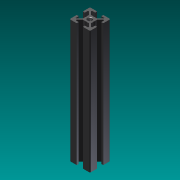
# Autodesk Inventor part: HFSY5-2020-120-TPW
Saved by Autodesk Inventor 2015 (Build 190159000, 159)
## iProperties
Category: PARTsolutions
Company: MISUMI
Created: 2016-02-29
Part Number: HFSY5-2020-120-TPW
Catalog Web Link: www.cadenas.de
Description: NFS5-2020, NFSB5-2020, HFS5-2020, HFSB5-2020, CAF5-2020, HFSY5-2020, NFSF5-2020, HFSF5-2020, HFSFB5-2020, NFST5-2020, HFST5-2020, HFSTB5-2020, HFSH5-2020, HFSC5-2020-HFS5 Series Aluminum Extrusions 20 Square -1 Slot-
Vendor: MISUMI
Document SubType Name: Modeling
Designer: psAdmin
Manufacturer: MISUMI
Mass: 21.8665 g
Surface Area: 212.07 cm^2
Volume: 21.8665 cm^3
Density: 1 g/cm^3
Material: 一般
Appearance: PSOLRGB-175-175-175
PSOL_IDENT_0: {$CADENAS_DATA\23d-libs\misumi\metric\38_al_extrusions_blackets\5\hfs5_2020.prj},580 {VTYP=3D},{NB=H
PSOL_IDENT_1: FSY5-2020-120-TPW},{LINA=HFSY5-2020-120-TPW},{NN=NFS5-2020, NFSB5-2020, HFS5-2020, HFSB5-2020, CAF5-
PSOL_IDENT_2: 2020, HFSY5-2020, NFSF5-2020, HFSF5-2020, HFSFB5-2020, NFST5-2020, HFST5-2020, HFSTB5-2020, HFSH5-20
PSOL_IDENT_3: 20, HFSC5-2020},{DATE=17.07.2015 10:47:07},{GEOMDATE=28.10.2014 00:00:00},{VERSION=},{LINEID=120},{L
PSOL_IDENT_4: INESUBID=-1},{WBVAR=L,ALT1,ALT2,ALT4,ALT5,CP5,DL5,DR5,ALT6,ALT9,ALT10,ALT11,HP6,NHL6,DL6,NHR6,DR6,AL
PSOL_IDENT_5: T7,ALT8,NH9,AH,BH,CH,DH,EH,NH10,AV,BV,CV,DV,EV,NH11,AP,BP,CP,DP,EP,ALT12,ALT13,Z,NH12,XA,XB,XC,XD,XE
PSOL_IDENT_6: ,NH13,YA,YB,YC,YD,YE,ALT16,HP16,DL16,DR16,ALT17,HQ17,JLP,ALT20}  {NB=HFSY5-2020-120-TPW},{LINA=HFSY5
PSOL_IDENT_7: -2020-120-TPW},{KT=DUMMY},{PN=HFSY5-2020-120-TPW},{TPS=HFSY5-2020},{MAT=A6N01SS-T5 Aluminum Alloy or
PSOL_IDENT_8: 6005A-T5 Aluminum Alloy},{ST=Baked-on Finish (Yellow)},{FRMW=20},{FRMH=20},{FRD=4.2},{L=120},{MASS=
PSOL_IDENT_9: 0.5},{SA=183},{LX=0.742x10^4},{LY=0.742x10^4},{ALT1=TPW},{M1=5},{DPL1=15},{DPR1=15},{ALT1PN=-TPW},{A
PSOL_IDENT_10: LT2=},{ALT2ALG= '','Not applicable' },{M2=0},{DP2=0},{ALT2PN=},{ALT4=},{ALT4ALG= '', 'w/o SC (High P
PSOL_IDENT_11: recision Cut)', 'SC', 'with SC (High Precision Cut)' },{ALT4PN=},{ALT5=},{ALT5ALG= '','w/o 45 Degree
PSOL_IDENT_12: Cut','1','with 45 Degree Cut' },{CP5=},{CP5ALG= '','N/A' },{DL5=},{DL5ALG= '','N/A' },{DR5=},{DR5AL
PSOL_IDENT_13: G= '','N/A' },{FRMLALT5=0},{FRMRALT5=0},{ALT5PN=},{ALT6=},{ALT6ALG= '','w/o Fastening Location Wrenc
PSOL_IDENT_14: h Access Hole Alterations','1','with Fastening Location Wrench Access Hole Alterations' },{ALT9=},{A
PSOL_IDENT_15: LT9ALG= '','w/o Location Specified Wrench Access Hole Alteratons (Horizontal)','1','with Location Sp
PSOL_IDENT_16: ecified Wrench Access Hole Alteratons (Horizontal)' },{ALT10=},{ALT10ALG= '','w/o Location Specified
PSOL_IDENT_17: Wrench Access Hole Alteratons (Vertical)','1','with Location Specified Wrench Access Hole Alteraton
PSOL_IDENT_18: s (Vertical)' },{ALT11=},{ALT11ALG= '','w/o Location Specified Wrench Access Hole Alteratons (Crissc
PSOL_IDENT_19: ross)','1','with Location Specified Wrench Access Hole Alteratons (Crisscross)' },{HP6=},{HP6ALG= ''
PSOL_IDENT_20: ,'N/A' },{NHL6=},{NHL6ALG= '','N/A' },{DL6=},{DL6ALG= '','N/A' },{NHR6=},{NHR6ALG= '','N/A' },{DR6=}
PSOL_IDENT_21: ,{DR6ALG= '','N/A' },{HL6=0},{HL6D=0},{HR6=0},{HR6D=0},{J6=0},{J6D=0},{K6=0},{K6D=0},{DD6=0.00},{DD6
PSOL_IDENT_22: ALG=0},{ALT7=},{ALT7ALG= '','N/A' },{ALT8=},{ALT8ALG= '','N/A' },{ALT678PN=},{NH9=0},{NH9MAX=5},{NH9
PSOL_IDENT_23: ALG=[0]},{AH=0.0},{AHMIN=7},{AHMAX=115},{AHALG=[0]},{BH=0.0},{BHMIN=2},{BHMAX=117},{BHALG=[0]},{CH=0
PSOL_IDENT_24: .0},{CHMIN=2},{CHMAX=119},{CHALG=[0]},{DH=0.0},{DHMIN=2},{DHMAX=121},{DHALG=[0]},{EH=0.0},{EHMIN=2},
PSOL_IDENT_25: {EHMAX=113},{EHALG=[0]},{NH10=0},{NH10MAX=5},{NH10ALG=[0]},{AV=0.0},{AVMIN=7},{AVMAX=115},{AVALG=[0]
PSOL_IDENT_26: },{BV=0.0},{BVMIN=2},{BVMAX=117},{BVALG=[0]},{CV=0.0},{CVMIN=2},{CVMAX=119},{CVALG=[0]},{DV=0.0},{DV
PSOL_IDENT_27: MIN=2},{DVMAX=121},{DVALG=[0]},{EV=0.0},{EVMIN=2},{EVMAX=113},{EVALG=[0]},{NH11=0},{NH11MAX=5},{NH11
PSOL_IDENT_28: ALG=[0]},{AP=0.0},{APMIN=7},{APMAX=115},{APALG=[0]},{BP=0.0},{BPMIN=2},{BPMAX=117},{BPALG=[0]},{CP=0
PSOL_IDENT_29: .0},{CPMIN=2},{CPMAX=119},{CPALG=[0]},{DP=0.0},{DPMIN=2},{DPMAX=121},{DPALG=[0]},{EP=0.0},{EPMIN=2},
PSOL_IDENT_30: {EPMAX=113},{EPALG=[0]},{ALT9PN=},{ALT10PN=},{ALT11PN=},{ALT91011PN=},{ALT12=},{ALT12ALG= '','w/o Co
PSOL_IDENT_31: unterbore Hole in Specified Position (Vertical)','1','with Counterbore Hole in Specified Position (V
PSOL_IDENT_32: ertical)' },{ALT13=},{ALT13ALG= '','w/o Counterbore Hole in Specified Position (Horizontal)','1','wi
PSOL_IDENT_33: th Counterbore Hole in Specified Position (Horizontal)' },{Z=},{ZALG= '','N/A' },{DD12=0.0},{DD112=0
PSOL_IDENT_34: .0},{NH12=0},{NH12MAX=5},{NH12ALG=[0]},{XA=0.0},{XAMIN=7},{XAMAX=115},{XAALG=[0]},{XB=0.0},{XBMIN=2}
PSOL_IDENT_35: ,{XBMAX=117},{XBALG=[0]},{XC=0.0},{XCMIN=2},{XCMAX=119},{XCALG=[0]},{XD=0.0},{XDMIN=2},{XDMAX=121},{
PSOL_IDENT_36: XDALG=[0]},{XE=0.0},{XEMIN=2},{XEMAX=113},{XEALG=[0]},{NH13=0},{NH13MAX=5},{NH13ALG=[0]},{YA=0.0},{Y
PSOL_IDENT_37: AMIN=7},{YAMAX=115},{YAALG=[0]},{YB=0.0},{YBMIN=2},{YBMAX=117},{YBALG=[0]},{YC=0.0},{YCMIN=2},{YCMAX=
PSOL_IDENT_38: 119},{YCALG=[0]},{YD=0.0},{YDMIN=2},{YDMAX=121},{YDALG=[0]},{YE=0.0},{YEMIN=2},{YEMAX=113},{YEALG=[0
PSOL_IDENT_39: ]},{ALT12PN=},{ALT13PN=},{ALT1213PN=},{ALT16=},{ALT16ALG= '','w/o M Type Hole Alteration','1','with
PSOL_IDENT_40: M Type Hole Alteration' },{HP16=},{HP16ALG= '','N/A' },{DL16=},{DL16ALG= '','N/A' },{DR16=},{DR16ALG=
PSOL_IDENT_41: '','N/A' },{H116=0},{D16=0.0},{ALT16PN=},{ALT17=},{ALT17ALG= '','w/o L Type Hole Alteration (Top)','
PSOL_IDENT_42: 1','with L Type Hole Alteration (Top)' },{HQ17=0},{HQ17ALG=0},{JLP=0},{JLPMIN=4.9},{JLPMAX=0},{JLPAL
PSOL_IDENT_43: G=[0]},{L17=0},{D17=0.0},{ALT17PN=},{ALT20=},{ALT20PN=},{ERRORALT01=OK},{ERRORALT02=OK},{ERRORALT05=
PSOL_IDENT_44: OK},{ERRORALT06091=OK},{ERRORALT06092=OK},{ERRORALT06093=OK},{ERRORALT06094=OK},{ERRORALT06101=OK},{
PSOL_IDENT_45: ERRORALT06102=OK},{ERRORALT06103=OK},{ERRORALT06104=OK},{ERRORALT06111=OK},{ERRORALT06112=OK},{ERROR
PSOL_IDENT_46: ALT06113=OK},{ERRORALT06114=OK},{ERRORALT06121=OK},{ERRORALT06122=OK},{ERRORALT06123=OK},{ERRORALT06
PSOL_IDENT_47: 124=OK},{ERRORALT06131=OK},{ERRORALT06132=OK},{ERRORALT06133=OK},{ERRORALT06134=OK},{ERRORALT0616=OK
PSOL_IDENT_48: },{ERRORALT06171=OK},{ERRORALT06172=OK},{ERRORALT06173=OK},{ERRORALT0911=OK},{ERRORALT0913=OK},{ERRO
PSOL_IDENT_49: RALT0916=OK},{ERRORALT0917=OK},{ERRORALT1011=OK},{ERRORALT1012=OK},{ERRORALT1016=OK},{ERRORALT1017=O
PSOL_IDENT_50: K},{ERRORALT1112=OK},{ERRORALT1113=OK},{ERRORALT1116=OK},{ERRORALT1117=OK},{ERRORALT1216=OK},{ERRORA
PSOL_IDENT_51: LT1217=OK},{ERRORALT1316=OK},{ERRORALT1317=OK},{ERRORALT1617=OK},{ERRORPN=},{TFW=0}
NN: NFS5-2020, NFSB5-2020, HFS5-2020, HFSB5-2020, CAF5-2020, HFSY5-2020, NFSF5-2020, HFSF5-2020, HFSFB5-2020, NFST5-2020, HFST5-2020, HFSTB5-2020, HFSH5-2020, HFSC5-2020
NT: HFS5 Series Aluminum Extrusions 20 Square -1 Slot-
NB: HFSY5-2020-120-TPW
NBSYN: $PN.
LINA: HFSY5-2020-120-TPW
PN: HFSY5-2020-120-TPW
TPS: HFSY5-2020
MAT: A6N01SS-T5 Aluminum Alloy or 6005A-T5 Aluminum Alloy
ST: Baked-on Finish (Yellow)
L: 120
MASS: 0.5
SA: 183
LX: 0.742x10^4
LY: 0.742x10^4
ALT1: with TPW (Tapping on Both Ends)
M1: 5
DPL1: 15
DPR1: 15
ALT2: Not applicable
M2: 0
DP2: 0
ALT4: w/o SC (High Precision Cut)
ALT5: w/o 45 Degree Cut
CP5: N/A
DL5: N/A
DR5: N/A
ALT6: w/o Fastening Location Wrench Access Hole Alterations
ALT9: w/o Location Specified Wrench Access Hole Alteratons (Horizontal)
ALT10: w/o Location Specified Wrench Access Hole Alteratons (Vertical)
ALT11: w/o Location Specified Wrench Access Hole Alteratons (Crisscross)
HP6: N/A
NHL6: N/A
DL6: N/A
NHR6: N/A
DR6: N/A
HL6D: 0
HR6D: 0
J6D: 0
K6D: 0
DD6: 0.00
ALT7: N/A
ALT8: N/A
NH9: 0
AH: 0.0
BH: 0.0
CH: 0.0
DH: 0.0
EH: 0.0
NH10: 0
AV: 0.0
BV: 0.0
CV: 0.0
DV: 0.0
EV: 0.0
NH11: 0
AP: 0.0
BP: 0.0
CP: 0.0
DP: 0.0
EP: 0.0
ALT12: w/o Counterbore Hole in Specified Position (Vertical)
ALT13: w/o Counterbore Hole in Specified Position (Horizontal)
Z: N/A
DD12: 0.0
DD112: 0.0
NH12: 0
XA: 0.0
XB: 0.0
XC: 0.0
XD: 0.0
XE: 0.0
NH13: 0
YA: 0.0
YB: 0.0
YC: 0.0
YD: 0.0
YE: 0.0
ALT16: w/o M Type Hole Alteration
HP16: N/A
DL16: N/A
DR16: N/A
H116: 0
D16: 0.0
ALT17: w/o L Type Hole Alteration (Top)
HQ17: 0
JLP: 0
D17: 0.0
ALT20: w/o CW (End Face C Chamfering)
SUPPLIER: MISUMI
ARTICLENO: HFSY5-2020-120-TPW
BOMINFO: HFSY5-2020-120-TPW
CREATOR: CADENAS GmbH
Title: HFSY5-2020-120-TPW
Author: Cadenas PARTsolutions
Comments: HFS5 Series Aluminum Extrusions 20 Square -1 Slot-
Autodesk Inventor part; units mm, degrees
sketch "Sketch_1" plane through (0, 0, 0) normal (0, 0, 1) x (1, 0, 0)
  line L0 (-10, 3) -> (-8, 3)
  line L1 (-8, 3) -> (-8, 6)
  line L2 (-8, 6) -> (-7.0607, 6)
  line L3 (-7.0607, 6) -> (-4, 2.9393)
  line L4 (-4, 2.9393) -> (-4, 0.5196)
  line L5 (-4, 0.5196) -> (-3.7, 0)
  line L6 (-3.7, 0) -> (-4, -0.5196)
  line L7 (-4, -0.5196) -> (-4, -2.9393)
  line L8 (-4, -2.9393) -> (-7.0607, -6)
  line L9 (-7.0607, -6) -> (-8, -6)
  line L10 (-8, -6) -> (-8, -3)
  line L11 (-8, -3) -> (-10, -3)
  line L12 (-10, -3) -> (-10, -9)
  arc A0 (-10, -9) -> (-9, -10) centre (-9, -9) ccw
  line L13 (-9, -10) -> (-3, -10)
  line L14 (-3, -10) -> (-3, -8)
  line L15 (-3, -8) -> (-6, -8)
  line L16 (-6, -8) -> (-6, -7.0607)
  line L17 (-6, -7.0607) -> (-2.9393, -4)
  line L18 (-2.9393, -4) -> (-0.5196, -4)
  line L19 (-0.5196, -4) -> (0, -3.7)
  line L20 (0, -3.7) -> (0.5196, -4)
  line L21 (0.5196, -4) -> (2.9393, -4)
  line L22 (2.9393, -4) -> (6, -7.0607)
  line L23 (6, -7.0607) -> (6, -8)
  line L24 (6, -8) -> (3, -8)
  line L25 (3, -8) -> (3, -10)
  line L26 (3, -10) -> (9, -10)
  arc A1 (9, -10) -> (10, -9) centre (9, -9) ccw
  line L27 (10, -9) -> (10, -3)
  line L28 (10, -3) -> (8, -3)
  line L29 (8, -3) -> (8, -6)
  line L30 (8, -6) -> (7.0607, -6)
  line L31 (7.0607, -6) -> (4, -2.9393)
  line L32 (4, -2.9393) -> (4, -0.5196)
  line L33 (4, -0.5196) -> (3.7, 0)
  line L34 (3.7, 0) -> (4, 0.5196)
  line L35 (4, 0.5196) -> (4, 2.9393)
  line L36 (4, 2.9393) -> (7.0607, 6)
  line L37 (7.0607, 6) -> (8, 6)
  line L38 (8, 6) -> (8, 3)
  line L39 (8, 3) -> (10, 3)
  line L40 (10, 3) -> (10, 9)
  arc A2 (10, 9) -> (9, 10) centre (9, 9) ccw
  line L41 (9, 10) -> (3, 10)
  line L42 (3, 10) -> (3, 8)
  line L43 (3, 8) -> (6, 8)
  line L44 (6, 8) -> (6, 7.0607)
  line L45 (6, 7.0607) -> (2.9393, 4)
  line L46 (2.9393, 4) -> (0.5196, 4)
  line L47 (0.5196, 4) -> (0, 3.7)
  line L48 (0, 3.7) -> (-0.5196, 4)
  line L49 (-0.5196, 4) -> (-2.9393, 4)
  line L50 (-2.9393, 4) -> (-6, 7.0607)
  line L51 (-6, 7.0607) -> (-6, 8)
  line L52 (-6, 8) -> (-3, 8)
  line L53 (-3, 8) -> (-3, 10)
  line L54 (-3, 10) -> (-9, 10)
  arc A3 (-9, 10) -> (-10, 9) centre (-9, 9) ccw
  line L55 (-10, 9) -> (-10, 3)
  constraints: 112 end point, 8 point on circle, 4 centre point
extrude "Extrusion1" add sketch "Sketch_1" against normal blind 120
sketch "Sketch2" plane through (0, 0, 0) normal (0, 0, 1) x (1, 0, 0)
  point P0 (0, 0)
hole "Hole1" at (0, 0, 0) direction (0, 0, -1) diameter 4.134 depth 15 countersink diameter 5 countersink angle 90 thread size "M5x0.8" class "6H" standard "ISO Metric profile"
sketch "Sketch3" plane through (0, 0, -120) normal (0, 0, -1) x (-1, 0, 0)
  point P0 (0, 0)
hole "Hole2" at (0, 0, -120) direction (0, 0, 1) diameter 4.134 depth 15 countersink diameter 5 countersink angle 90 thread size "M5x0.8" class "6H" standard "ISO Metric profile"
sketch "Sketch4" plane through (0, 0, -105) normal (0, 0, -1) x (-1, 0, 0)
  point P0 (0, 0)
hole "Hole3" at (0, 0, -105) direction (0, 0, 1) diameter 4.2 depth 90
ref_plane "C1_XY" through (0, 0, 0) normal (0, 0, 1) x (1, 0, 0)
ref_plane "C1_YZ" through (0, 0, 0) normal (1, 0, 0) x (0, 1, 0)
ref_plane "C1_ZX" through (0, 0, 0) normal (0, 1, 0) x (0, 0, 1)
body "Solid1"
